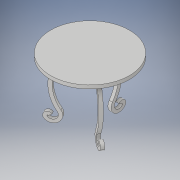
# Autodesk Inventor part: table round
Saved by Autodesk Inventor 2017 (Build 210142000, 142)
## iProperties
Created: 2018-03-05
Part Number: table round
Material: Generic
Document SubType Name: Modeling
Designer: Braxton
Density: 1 g/cm^3
Appearance: Default
Author: Braxton
Autodesk Inventor part; units mm, degrees
ref_plane "YZ Plane" through (0, 0, 0) normal (1, 0, 0) x (0, 1, 0)
ref_plane "XZ Plane" through (0, 0, 0) normal (0, 1, 0) x (-1, 0, 0)
ref_plane "XY Plane" through (0, 0, 0) normal (0, 0, 1) x (1, 0, 0)
sketch "Sketch1" plane through (0, 0, 0) normal (1, 0, 0) x (0, 1, 0)
  arc A0 (0.7409, -6.9281) -> (1.6287, -5.6125) centre (1.1834, -6.2693) ccw
  line L0 (1.6287, -5.6125) -> (1.2582, -6.1591)
  line L1 (0.7409, -6.9281) -> (1.1092, -6.3799) construction
  line L2 (2.519, -4.2812) -> (2.1507, -4.8294) construction
  arc A1 (1.1092, -6.3799) -> (1.2582, -6.1591) centre (1.1834, -6.2693) ccw
  arc A2 (2.1507, -4.8294) -> (1.1092, -6.3799) centre (1.63, -5.6046) ccw
  arc A3 (2.1507, -4.8294) -> (12.3205, -4.2899) centre (6.8767, 2.206) ccw
  arc A4 (2.519, -4.2812) -> (11.8963, -3.7838) centre (6.8767, 2.206) ccw
  arc A5 (12.3205, -4.2899) -> (12.9142, -3.0177) centre (11.2543, -3.0177) ccw
  arc A6 (11.8963, -3.7838) -> (12.2538, -3.0177) centre (11.2543, -3.0177) ccw
  line L3 (11.8963, -3.7838) -> (12.3205, -4.2899) construction
  line L4 (12.2538, -3.0177) -> (12.9142, -3.0177) construction
  arc A7 (12.2538, -3.0177) -> (10.7251, -3.0177) centre (11.4895, -3.0177) ccw
  line L5 (10.7251, -3.0177) -> (10.0647, -3.0177)
  arc A8 (12.9142, -3.0177) -> (10.0647, -3.0177) centre (11.4895, -3.0177) ccw
  line L6 (0.0665, -5.2922) -> (0.0665, -5.917)
  arc A9 (2.519, -4.2812) -> (0.0665, -5.2922) centre (1.63, -5.6046) ccw
  arc A10 (0.0665, -5.917) -> (0.7409, -6.9281) centre (1.63, -5.6046) ccw
  point P0 (0, 0)
  point P1 (12.584, -3.0177)
  dimension "d10" = 0.6604
  dimension "d11" = 0.6604
  dimension "d12" = 0.6604
  dimension "d15" = 0.6604
  constraints: 22 point on circle, 14 end point, 11 centre point, 5 line through centre, 5 tangent, 2 concentric, 1 horizontal, 1 midpoint, 1 point on line, 1 vertical, 2 other
  measures "d10" distance of L0.start L0.end
  measures "d11" distance of L1.start L1.end
  measures "d12" distance of L2.start L2.end
  measures "d15" distance of L5.start L5.end
extrude "leg" add sketch "Sketch1" along normal mid plane 0.6604
pattern_circular "Circular Pattern1" count 3 over 360 about axis through (0, -10, 0) along (0, 1, 0) of "leg"
sketch "Sketch2" plane through (0, 0, 0) normal (1, 0, 0) x (0, 1, 0)
  arc A0 (11.8963, -3.7838) -> (12.2538, -3.0177) centre (11.2543, -3.0177) ccw projected
  arc A1 (12.3205, -4.2899) -> (12.9142, -3.0177) centre (11.2543, -3.0177) ccw projected
  arc A2 (11.8963, -3.7838) -> (12.2538, -3.0177) centre (11.2543, -3.0177) ccw projected
  line L0 (12.2538, -3.0177) -> (12.9142, -3.0177)
  line L1 (12.584, -3.0177) -> (13.2952, -3.0177) construction
  line L2 (13.2952, -3.0177) -> (13.2952, 0.0049)
  line L3 (13.2952, 0.0049) -> (12.584, 0.0049)
  line L4 (12.584, 0.0049) -> (12.584, -3.0177)
  line L5 (13.2952, -3.0177) -> (13.2952, -8.0977)
  line L6 (13.2952, -8.0977) -> (12.584, -8.0977)
  line L7 (12.584, -8.0977) -> (12.584, -3.0177)
  point P0 (0, 0)
  dimension "d21" = 0.7112
  dimension "d22" = 3.0226
  dimension "d23" = 5.08
  constraints: 16 end point, 5 perpendicular, 1 horizontal, 1 midpoint, 1 point on line, 1 vertical
  measures "d21" distance of L1.start L1.end
  measures "d22" distance of L1.end L2.end
  measures "d23" distance of L1.end L5.end
revolve "Revolution1" add sketch "Sketch2" angle 360 about axis through (0, 13.2952, 0.0049) along (0, -1, 0)
body "Solid1"
